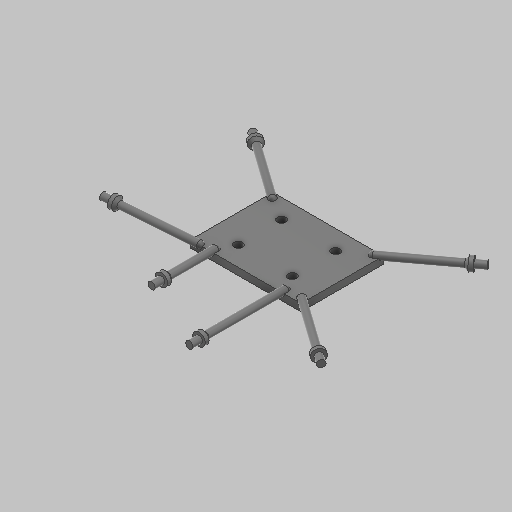
# Autodesk Inventor part: MARCADOR_ROBOTAT
Saved by Autodesk Inventor 2024.2 (Build 282272000, 272)
## iProperties
Created: 2023-10-04
Part Number: MARCADOR_ROBOTAT
Material: ABS Plastic
Document SubType Name: Modeling
Designer: jalva
Density: 1.06 g/cm^3
Appearance: Smooth - White
Mass: 8.91175 g
Surface Area: 70.9966 cm^2
Volume: 8.40731 cm^3
Author: jalva
Autodesk Inventor part; units mm, degrees
sketch "Sketch1" plane through (0, 0, 0) normal (0, 1, 0) x (-1, 0, 0)
  line L0 (25.5, 19) -> (-25.5, 19)
  line L1 (-25.5, 19) -> (-25.5, -19)
  line L2 (-25.5, -19) -> (25.5, -19)
  line L3 (25.5, -19) -> (25.5, 19)
  line L4 (25.5, 19) -> (-25.5, -19) construction
  line L5 (-25.5, 19) -> (25.5, -19) construction
  line L6 (12.5, 10) -> (-12.5, 10) construction
  line L7 (-12.5, 10) -> (-12.5, -10) construction
  line L8 (-12.5, -10) -> (12.5, -10) construction
  line L9 (12.5, -10) -> (12.5, 10) construction
  line L10 (12.5, 10) -> (-12.5, -10) construction
  line L11 (-12.5, 10) -> (12.5, -10) construction
  circle A0 centre (-12.5, -10) radius 2
  circle A1 centre (-12.5, 10) radius 2
  circle A2 centre (12.5, 10) radius 2
  circle A3 centre (12.5, -10) radius 2
  point P0 (0, 0)
  dimension "d0" = 38
  dimension "d1" = 51
  dimension "d2" = 25
  dimension "d3" = 20
  dimension "d4" = 4
  constraints: 24 end point, 4 centre point, 4 coincident, 4 midpoint, 4 parallel, 3 equal radius, 2 horizontal, 2 perpendicular
  measures "d0" distance of L0.end L1.end
  measures "d1" distance between parallel lines of L3 L1
  measures "d2" distance of L7.end L8.end
  measures "d3" distance of L6.end L7.end
  measures "d4" diameter of A0
extrude "Extrusion1" add sketch "Sketch1" along normal blind 3.3
sketch "Sketch2" plane through (0, 3.3, 0) normal (0, 1, 0) x (1, 0, 0)
  line L0 (21.4906, 16.0126) -> (53.217, 39.6519)
  line L1 (25.5, -19) -> (25.5, 19) construction
  line L2 (0, 0) -> (25.5, 19) construction
  dimension "d7" = 5
  constraints: 4 end point, 1 collinear, 1 point on line
  measures "d7" distance of L1.end L0.start
ref_plane "Work Plane1" through (53.217, 3.3, -39.6519) normal (0.8018828, 0, -0.5974813) x (0, 1, 0)
sketch "Sketch3" plane through (53.217, 3.3, -39.6519) normal (0.8018828, 0, -0.5974813) x (0, 1, 0)
  circle A0 centre (0, 0) radius 1.65
  point P0 (-3.3, 0)
  point P1 (0, 0)
  dimension "d8" = 3.3
  constraints: 1 centre point, 1 coincident
  measures "d8" diameter of A0
sweep "Sweep1" add profiles "Sketch3" path "Sketch2"
fillet "Fillet1" radius 1.65 2 edges at (20.7935, 4.4667, -16.9482) (22.1877, 4.4667, -15.077)
ref_plane "Work Plane2" through (49.6086, 3.3, -36.9632) normal (0.8018828, 0, -0.5974813) x (0, 1, 0)
sketch "Sketch4" plane through (49.6086, 3.3, -36.9632) normal (0.8018828, 0, -0.5974813) x (0, 1, 0)
  circle A0 centre (0, 0) radius 2.9
  circle A1 centre (0, 0) radius 1.65 projected
  point P0 (-3.3, 0)
  dimension "d19" = 5.8
  constraints: 1 centre point, 1 coincident
  measures "d19" diameter of A0
extrude "Extrusion2" add sketch "Sketch4" against normal blind 3
chamfer "Chamfer1" distance 1.25 angle 45 1 edges at (47.2029, 0.4, -35.1708)
pattern_circular "Circular Pattern1" count 2 over 108 about axis through (0, -10, 0) along (0, 1, 0) of "Sweep1", "Fillet1", "Extrusion2", "Chamfer1"
pattern_circular "Circular Pattern2" count 2 over 72 about axis through (0, -10, 0) along (0, -1, 0) of "Sweep1", "Fillet1", "Extrusion2", "Chamfer1"
sketch "Sketch5" plane through (0, 3.3, 0) normal (0, 1, 0) x (1, 0, 0)
  circle A0 centre (12.5, -10) radius 2 projected
  line L0 (16.2, -61.3) -> (16.2, -15.3)
  line L1 (-25.5, -19) -> (23.9698, -19) projected
  point P0 (0, 0)
  dimension "d25" = 3.7
  dimension "d26" = 3.7
  dimension "d27" = 46
  constraints: 2 end point, 1 vertical
  measures "d25" distance from line of L0 A0.centre
  measures "d26" distance from line of L1 L0.end
  measures "d27" distance of L0.start L0.end
ref_plane "Work Plane3" through (16.2, 3.3, 61.3) normal (0, 0, -1) x (-1, 0, 0)
sketch "Sketch6" plane through (16.2, 3.3, 61.3) normal (0, 0, -1) x (-1, 0, 0)
  circle A0 centre (0, 0) radius 1.65
  point P0 (16.2, -3.3)
  dimension "d28" = 3.3
  constraints: 1 centre point, 1 coincident
  measures "d28" diameter of A0
sweep "Sweep2" add profiles "Sketch6" path "Sketch5" path curves L0
fillet "Fillet2" radius 1.65 1 edges at (16.2, 4.95, 15.3)
ref_plane "Work Plane5" through (16.2, 3.3, 56.8) normal (0, 0, -1) x (-1, 0, 0)
sketch "Sketch7" plane through (16.2, 3.3, 56.8) normal (0, 0, -1) x (-1, 0, 0)
  circle A0 centre (0, 0) radius 1.65 projected
  circle A1 centre (0, 0) radius 2.9
  point P0 (16.2, -3.3)
  dimension "d34" = 5.8
  constraints: 1 centre point, 1 coincident
  measures "d34" diameter of A1
extrude "Extrusion3" add sketch "Sketch7" along normal blind 3
chamfer "Chamfer2" distance 1.25 angle 45 1 edges at (19.1, 3.3, 53.8)
sketch "Sketch8" plane through (0, 3.3, 0) normal (0, 1, 0) x (1, 0, 0)
  circle A0 centre (-12.5, -10) radius 2 projected
  line L0 (-16.2, -15.3) -> (-16.2, -46.3)
  line L1 (-25.5, -19) -> (14.55, -19) projected
  point P0 (0, 0)
  dimension "d40" = 3.7
  dimension "d41" = 3.7
  dimension "d42" = 31
  constraints: 2 end point, 1 vertical
  measures "d40" distance from line of A0.centre L0
  measures "d41" distance from line of L1 L0.start
  measures "d42" distance of L0.start L0.end
ref_plane "Work Plane6" through (-16.2, 3.3, 46.3) normal (0, 0, 1) x (1, 0, 0)
sketch "Sketch9" plane through (-16.2, 3.3, 46.3) normal (0, 0, 1) x (1, 0, 0)
  circle A0 centre (0, 0) radius 1.65
  point P0 (16.2, -3.3)
  dimension "d43" = 3.3
  constraints: 1 centre point, 1 coincident
  measures "d43" diameter of A0
sweep "Sweep3" add profiles "Sketch9" path "Sketch8" path curves L0
fillet "Fillet3" radius 1.65 1 edges at (-16.2, 4.95, 15.3)
ref_plane "Work Plane7" through (-16.2, 3.3, 41.8) normal (0, 0, 1) x (1, 0, 0)
sketch "Sketch10" plane through (-16.2, 3.3, 41.8) normal (0, 0, 1) x (1, 0, 0)
  circle A0 centre (0, 0) radius 2.9
  circle A1 centre (0, 0) radius 1.65 projected
  point P0 (16.2, -3.3)
  dimension "d48" = 5.8
  constraints: 1 centre point, 1 coincident
  measures "d48" diameter of A0
extrude "Extrusion4" add sketch "Sketch10" against normal blind 3
chamfer "Chamfer3" distance 1.25 angle 45 1 edges at (-19.1, 3.3, 38.8)
sketch "Sketch11" plane through (0, 3.3, 0) normal (0, 1, 0) x (1, 0, 0)
  line L0 (-25.5, -19) -> (21.8698, -15.4906) construction
  arc A0 (24.17, -15.0978) -> (22.2626, -17.7908) centre (23.2163, -16.4443) ccw projected
  line L1 (-20.05, -18.5962) -> (-63.2317, -21.7954)
  line L2 (-25.5, 16.0399) -> (-25.5, -19) projected
  point P0 (0, 0)
  dimension "d54" = 5.45
  dimension "d55" = 43.3
  constraints: 4 end point, 1 coincident, 1 collinear, 1 point on circle, 1 point on line
  measures "d54" distance from line of L2 L1.start
  measures "d55" distance of L1.start L1.end
ref_plane "Work Plane8" through (-63.2317, 3.3, 21.7954) normal (-0.9972669, 0, 0.0738827) x (0, -1, 0)
sketch "Sketch12" plane through (-63.2317, 3.3, 21.7954) normal (-0.9972669, 0, 0.0738827) x (0, -1, 0)
  circle A0 centre (0, 0) radius 1.65
  point P0 (3.3, -17.0641)
  dimension "d56" = 3.3
  constraints: 1 centre point, 1 coincident
  measures "d56" diameter of A0
sweep "Sweep4" add profiles "Sketch12" path "Sketch11" path curves L1
fillet "Fillet4" radius 1.6 1 edges at (-19.9751, 4.602, 19.607)
ref_plane "Work Plane9" through (-58.744, 3.3, 21.4629) normal (-0.9972669, 0, 0.0738827) x (0, -1, 0)
sketch "Sketch13" plane through (-58.744, 3.3, 21.4629) normal (-0.9972669, 0, 0.0738827) x (0, -1, 0)
  circle A0 centre (0, 0) radius 1.65 projected
  arc A1 (1.625, 0.2863) -> (0, -1.65) centre (0, 0) ccw projected
  arc A2 (0, -1.65) -> (1.65, 0) centre (0, 0) ccw projected
  arc A3 (1.65, 0) -> (1.625, 0.2863) centre (0, 0) ccw projected
  circle A4 centre (0, 0) radius 2.9
  point P0 (3.3, -17.0641)
  dimension "d61" = 5.8
  constraints: 1 centre point, 1 coincident
  measures "d61" diameter of A4
extrude "Extrusion5" add sketch "Sketch13" against normal blind 3
chamfer "Chamfer4" distance 1.25 angle 45 1 edges at (-55.7522, 6.2, 21.2412)
body "Solid1"
